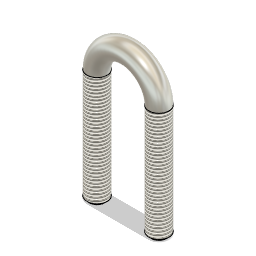
0.880.2544 - Etrier de 12-36-65 - VZC 21400_17 Rep. 90 (Autodesk Fusion 360 design; units mm, degrees)
Autodesk Fusion 360 part; units mm, degrees
sketch "Sketch1" plane through (0, 0, 0) normal (0, 0, 1) x (1, 0, 0)
  circle A0 centre (0, 0) radius 18 construction
  line L0 (0, 0) -> (50, 0) construction
  line L1 (0, 0) -> (0, 50) construction
  line L2 (0, 0) -> (-50, 0) construction
  line L3 (0, 0) -> (0, -100) construction
  line L4 (-18, 0) -> (-18, -65)
  line L5 (18, 0) -> (18, -65)
  arc A1 (18, 0) -> (-18, 0) centre (0, 0) ccw
  dimension "d1" = 36
  dimension "d6" = 65
  dimension "d7" = 65
  constraint coincident A0.centre L0.start
  constraint horizontal L0
  constraint vertical L1
  constraint horizontal L2
  constraint vertical L3
  constraint coincident L2 L4.start
  constraint coincident A0 L4.start
  constraint coincident A0 L5.start
  constraint coincident L0 L5.start
  constraint vertical L5
  constraint vertical L4
  measures "d1" diameter of A0
  measures "d6" distance of L4.start L4.end
  measures "d7" distance of L5.start L5.end
sketch "Sketch2" plane through (0, 0, 0) normal (0, 1, 0) x (1, 0, 0)
  circle A0 centre (18, 0) radius 6
  point P0 (18, 0)
  dimension "d8" = 12
  constraint coincident P0 A0.centre
  measures "d8" diameter of A0
sweep "Sweep1" add profiles "Sketch2" path "Sketch1" along L5 A1 L4 section 1
chamfer "Chamfer1" distance 1.5 angle 45 2 edges at (-12.406, -65, 2.1697) (12.406, -65, -2.1697)
thread "Thread1" "ISO Metric profile 12.0 M12x1.75 6g" major diameter 11.8335 minor diameter 9.8365 pitch 1.75 angle 60 resizes the face on face at (-23.9925, -42.3333, -0.2991)
thread "Thread2" "ISO Metric profile 12.0 M12x1.75 6g" major diameter 11.8335 minor diameter 9.8365 pitch 1.75 angle 60 resizes the face on face at (23.8873, -42.3888, -0.5891)
